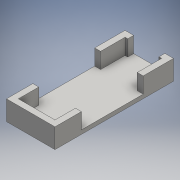
# Autodesk Inventor part: tapaArduino
Saved by Autodesk Inventor 2016 (Build 200138000, 138)
## iProperties
Created: 2016-04-24
Part Number: tapaArduino
Material: Generic
Document SubType Name: Modeling
Designer: Freddy Chang
Density: 1 g/cm^3
Appearance: Default
Author: Freddy Chang
Autodesk Inventor part; units mm, degrees
ref_plane "YZ Plane" through (0, 0, 0) normal (1, 0, 0) x (0, 1, 0)
ref_plane "XZ Plane" through (0, 0, 0) normal (0, 1, 0) x (-1, 0, 0)
ref_plane "XY Plane" through (0, 0, 0) normal (0, 0, 1) x (1, 0, 0)
sketch "Sketch1" plane through (0, 0, 0) normal (0, 0, 1) x (1, 0, 0)
  line L0 (0, 0) -> (24.55, 0)
  line L1 (24.55, 0) -> (24.55, -60)
  line L2 (24.55, -60) -> (0, -60)
  line L3 (0, -60) -> (0, 0)
  dimension "d0" = 24.55
  dimension "d1" = 60
  constraints: 8 end point, 2 parallel, 1 horizontal, 1 perpendicular
  measures "d0" distance of L1.end L2.end
  measures "d1" distance of L0.end L1.end
extrude "Extrusion1" add sketch "Sketch1" along normal blind 10
sketch "Sketch2" plane through (0, 0, 10) normal (0, 0, 1) x (1, 0, 0)
  line L0 (24.55, 0) -> (0, 0) projected
  line L1 (3, -3) -> (21.55, -3)
  line L2 (21.55, -3) -> (21.55, -57)
  line L3 (21.55, -57) -> (3, -57)
  line L4 (3, -57) -> (3, -3)
  line L5 (0, -60) -> (24.55, -60) projected
  line L6 (24.55, -60) -> (24.55, 0) projected
  line L7 (0, 0) -> (0, -60) projected
  dimension "d8" = 3
  dimension "d9" = 3
  dimension "d10" = 3
  dimension "d11" = 3
  constraints: 8 end point, 2 parallel, 1 horizontal, 1 perpendicular
  measures "d8" distance between parallel lines of L0 L1
  measures "d9" distance between parallel lines of L5 L3
  measures "d10" distance between parallel lines of L6 L2
  measures "d11" distance between parallel lines of L7 L4
extrude "Extrusion2" cut sketch "Sketch2" against normal blind 8 contours L1 L2 L3 L4
sketch "Sketch3" plane through (24.55, -60, 0) normal (1, 0, 0) x (0, 0, -1)
  line L0 (-10, 44.65) -> (-2, 44.65)
  line L1 (-2, 3) -> (-2, 57) projected
  line L2 (-10, 13.35) -> (-2, 13.35)
  line L3 (-2, 13.35) -> (-2, 44.65)
  line L4 (-10, 13.35) -> (-10, 44.65)
  line L5 (-10, 3) -> (-10, 57) projected
  line L6 (0, 60) -> (-10, 60) projected
  line L7 (0, 0) -> (-10, 0) projected
  dimension "d16" = 8
  dimension "d18" = 15.35
  dimension "d19" = 13.35
  constraints: 8 end point, 2 collinear, 2 point on line
  measures "d16" distance between parallel lines of L1 L4
  measures "d18" distance between parallel lines of L6 L0
  measures "d19" distance between parallel lines of L7 L2
extrude "Extrusion3" cut sketch "Sketch3" against normal blind 24.55
sketch "Sketch4" plane through (0, 0, 0) normal (0, 1, 0) x (1, 0, 0)
  line L0 (4.375, -10) -> (4.375, -2)
  line L1 (21.55, -2) -> (3, -2) projected
  line L2 (4.375, -2) -> (20.175, -2)
  line L3 (20.175, -2) -> (20.175, -10)
  line L4 (20.175, -10) -> (4.375, -10)
  line L5 (24.55, 0) -> (24.55, -10) projected
  point P0 (0, 0)
  dimension "d23" = 15.8
  dimension "d24" = 4.375
  dimension "d25" = 8
  dimension "d26" = 15.8
  constraints: 8 end point, 2 point on line, 1 horizontal, 1 perpendicular
  measures "d23" distance of L0.end L2.end
  measures "d24" distance between parallel lines of L5 L3
  measures "d25" distance of L0.start L0.end
  measures "d26" distance of L3.end L0.start
extrude "Extrusion4" cut sketch "Sketch4" against normal blind 3
body "Solid1"
